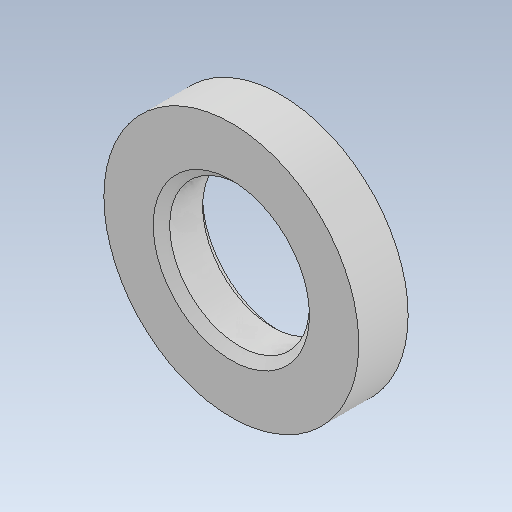
# Autodesk Inventor part: wheel_shift_1
Saved by Autodesk Inventor 2020 (Build 240168000, 168)
## iProperties
Created: 2020-05-15
Part Number: wheel_shift_1
Material: Generic
Document SubType Name: Modeling
Designer: psrobotics
Density: 1 g/cm^3
Appearance: Default
Author: psrobotics
Autodesk Inventor part; units mm, degrees
ref_plane "YZ Plane" through (0, 0, 0) normal (1, 0, 0) x (0, 1, 0)
ref_plane "XZ Plane" through (0, 0, 0) normal (0, 1, 0) x (-1, 0, 0)
sketch "Sketch1" plane through (0, 0, 0) normal (0, 0, 1) x (1, 0, 0)
  circle A0 centre (0, 0) radius 4 projected
  circle A1 centre (0, 0) radius 4.25
  circle A2 centre (0, 0) radius 7.75
  point P0 (0, 0)
  dimension "d0" = 8.5
  dimension "d1" = 15.5
  constraints: 2 centre point, 2 coincident
  measures "d0" diameter of A1
  measures "d1" diameter of A2
ref_plane "Work Plane1" through (-84.8968, -81.372, 3) normal (0, 0, -1) x (-0.5028459, 0.8643761, 0)
extrude "Extrusion1" add sketch "Sketch1" along normal up to surface (3 mm away) contours A2
chamfer "Chamfer1" distance 0.5 angle 45 2 edges at (-4.25, 0, 3) (-4.25, 0, 0)
body "Solid1"
